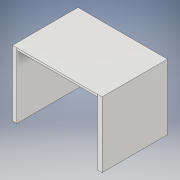
# Autodesk Inventor part: MAN_BASIS_THIRD_STRUCTURE
Saved by Autodesk Inventor 2019 (Build 230136000, 136)
## iProperties
Created: 2021-03-07
Part Number: MAN_BASIS_THIRD_STRUCTURE
Material: ABS Plastic
Document SubType Name: Modeling
Designer: DOMEK
Density: 1.06 g/cm^3
Appearance: Smooth - White
Author: DOMEK
Autodesk Inventor part; units mm, degrees
ref_plane "YZ Plane" through (0, 0, 0) normal (1, 0, 0) x (0, 1, 0)
ref_plane "XZ Plane" through (0, 0, 0) normal (0, 1, 0) x (-1, 0, 0)
ref_plane "XY Plane" through (0, 0, 0) normal (0, 0, 1) x (1, 0, 0)
sketch "Sketch1" plane through (0, 0, 0) normal (0, 1, 0) x (-1, 0, 0)
  line L0 (0, 0) -> (37, 0)
  line L1 (37, 0) -> (37, 30)
  line L2 (37, 30) -> (0, 30)
  line L3 (0, 30) -> (0, 0)
  dimension "d0" = 37
  dimension "d1" = 30
  constraints: 8 end point, 2 parallel, 1 horizontal, 1 perpendicular
  measures "d0" distance of L2.end L1.end
  measures "d1" distance of L1.end L0.end
extrude "Extrusion1" add sketch "Sketch1" along normal blind 1
sketch "Sketch2" plane through (0, 1, 0) normal (0, 1, 0) x (1, 0, 0)
  line L0 (-37, 0) -> (-37, -30) projected
  line L1 (-37, 0) -> (-39, 0)
  line L2 (-39, 0) -> (-39, -30)
  line L3 (-39, -30) -> (-37, -30)
  line L4 (-37, -30) -> (-37, 0)
  line L5 (0, 0) -> (-37, 0) projected
  line L6 (0, 0) -> (2, 0)
  line L7 (2, 0) -> (2, -30)
  line L8 (2, -30) -> (0, -30)
  line L9 (0, -30) -> (0, 0)
  dimension "d4" = 2
  dimension "d5" = 2
  constraints: 16 end point, 4 parallel, 2 horizontal, 2 perpendicular, 1 point on line
  measures "d4" distance of L3.end L2.end
  measures "d5" distance of L7.end L8.end
extrude "Extrusion2" add sketch "Sketch2" against normal blind 30
body "Solid1"
